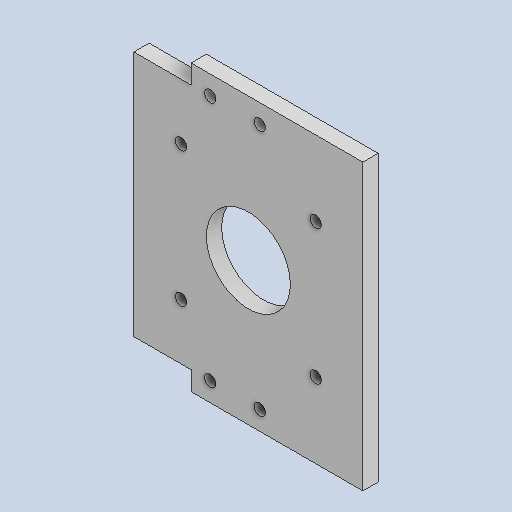
# Autodesk Inventor part: MotorHolder
Saved by Autodesk Inventor 2023 (Build 270158000, 158)
## iProperties
Created: 2024-02-03
Part Number: MotorHolder
Material: Generic
Document SubType Name: Modeling
Designer: victo
Density: 1 g/cm^3
Appearance: Default
Author: victo
Autodesk Inventor part; units mm, degrees
ref_plane "YZ Plane" through (0, 0, 0) normal (1, 0, 0) x (0, 1, 0)
ref_plane "XZ Plane" through (0, 0, 0) normal (0, 1, 0) x (-1, 0, 0)
ref_plane "XY Plane" through (0, 0, 0) normal (0, 0, 1) x (1, 0, 0)
sketch "Sketch1" plane through (0, 0, 0) normal (0, 0, 1) x (1, 0, 0)
  circle A0 centre (0, 0) radius 11
  line L0 (-15, 37.3) -> (30, 37.3)
  line L1 (30, 37.3) -> (30, -37.3)
  line L2 (30, -37.3) -> (-15, -37.3)
  line L3 (-15, -37.3) -> (-15, 37.3)
  line L4 (-15, 32.3) -> (-30, 32.3)
  line L5 (-30, 32.3) -> (-30, -32.3)
  line L6 (-30, -32.3) -> (-15, -32.3)
  line L7 (-15, -32.3) -> (-15, 32.3)
  circle A1 centre (-10, 32.3) radius 1.5
  circle A2 centre (3, 32.3) radius 1.5
  circle A3 centre (-10, -32.3) radius 1.5
  circle A4 centre (3, -32.3) radius 1.5
  circle A5 centre (-17.6398, 17.6398) radius 1.5
  line L8 (0, 0) -> (-17.6398, 17.6398) construction
  line L9 (0, 0) -> (-30, 0) construction
  circle A6 centre (-17.6398, -17.6398) radius 1.5
  circle A7 centre (17.6398, -17.6398) radius 1.5
  circle A8 centre (17.6398, 17.6398) radius 1.5
  point P0 (-15, -32.3)
  dimension "d0" = 22
  dimension "d1" = 3
  dimension "d2" = 3
  dimension "d3" = 3
  dimension "d4" = 3
  dimension "d5" = 5
  dimension "d6" = 5
  dimension "d7" = 5
  dimension "d8" = 13
  dimension "d9" = 13
  dimension "d10" = 5
  dimension "d11" = 5
  dimension "d12" = 5
  dimension "d13" = 74.6
  dimension "d14" = 37.3
  dimension "d15" = 60
  dimension "d16" = 15
  dimension "d17" = 5
  dimension "d18" = 5
  dimension "d19" = 30
  dimension "d20" = 3
  dimension "d22" = 45
  dimension "d25" = 360
  constraints: 20 end point, 9 centre point, 4 parallel, 2 horizontal, 2 perpendicular, 1 coincident, 1 midpoint, 1 point on line, 9 other
  measures "d0" diameter of A0
  measures "d1" diameter of A1
  measures "d2" diameter of A2
  measures "d3" diameter of A3
  measures "d4" diameter of A4
  measures "d5" distance from line of L3 A1.centre
  measures "d6" distance from line of L0 A1.centre
  measures "d7" distance from line of L0 A2.centre
  measures "d8" distance of A1.centre A2.centre
  measures "d9" distance of A4.centre A3.centre
  measures "d10" distance from line of L2 A3.centre
  measures "d11" distance from line of L2 A4.centre
  measures "d12" distance from line of L3 A3.centre
  measures "d13" distance between parallel lines of L2 L0
  measures "d14" distance from line of L0 point (0, 0)
  measures "d15" distance between parallel lines of L5 L1
  measures "d16" distance of L5.end L6.end
  measures "d17" distance between parallel lines of L2 L6
  measures "d18" distance between parallel lines of L0 L4
  measures "d19" distance from line of point (0, 0) L1
  measures "d20" diameter of A5
  measures "d22" angle of L9 L8
extrude "Extrusion1" add sketch "Sketch1" along normal blind 4
equation "\"d7\" = d6"
equation "\"d9\" = d8"
equation "\"d11\" = d10"
equation "\"d12\" = d10"
equation "\"d14\" = 0.5 * d13"
equation "\"d18\" = d17"
equation "\"d19\" = 0.5 * d15"
body "Solid1"
